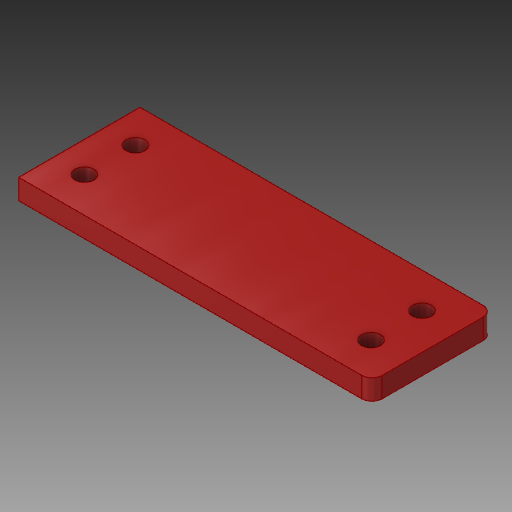
# Autodesk Inventor part: Gantry Chain Support
Saved by Autodesk Inventor 2019 (Build 230136000, 136)
## iProperties
Created: 2018-01-22
Part Number: Gantry Chain Support
Material: Steel
Document SubType Name: Modeling
Designer: torba
Density: 7.85 g/cm^3
Appearance: Red
Author: torba
Autodesk Inventor part; units mm, degrees
ref_plane "YZ Plane" through (0, 0, 0) normal (1, 0, 0) x (0, 1, 0)
ref_plane "XZ Plane" through (0, 0, 0) normal (0, 1, 0) x (-1, 0, 0)
ref_plane "XY Plane" through (0, 0, 0) normal (0, 0, 1) x (1, 0, 0)
sketch "Sketch1" plane through (0, 0, 0) normal (0, 1, 0) x (-1, 0, 0)
  circle A0 centre (-99.6006, 11.05) radius 3
  circle A1 centre (-9.6006, 11.05) radius 3
  circle A2 centre (-9.6006, 27.05) radius 3
  circle A3 centre (-99.6006, 27.05) radius 3
  arc A4 (-110.9506, 3.175) -> (-107.7756, 0) centre (-107.7756, 3.175) ccw
  line L0 (-107.7756, 0) -> (0, 0)
  line L1 (0, 38.1) -> (0, 0)
  line L2 (-107.7756, 38.1) -> (0, 38.1)
  arc A5 (-107.7756, 38.1) -> (-110.9506, 34.925) centre (-107.7756, 34.925) ccw
  line L3 (-110.9506, 3.175) -> (-110.9506, 34.925)
  point P0 (-62.2062, 0)
  dimension "d0" = 6
  dimension "d1" = 3.175
  dimension "d2" = 110.9506
  dimension "d3" = 38.1
  dimension "d4" = 0
  dimension "d5" = 38.1
  dimension "d6" = 9.6006
  dimension "d7" = 11.05
  dimension "d8" = 9.6006
  dimension "d9" = 27.05
  dimension "d10" = 62.2062
  dimension "d11" = 38.1
  dimension "d12" = 99.6006
  dimension "d13" = 11.05
  dimension "d14" = 99.6006
  dimension "d15" = 27.05
  constraints: 8 end point, 6 centre point, 4 equal radius, 4 point on circle, 4 tangent, 2 parallel, 1 horizontal, 1 vertical
  measures "d0" diameter of A2
  measures "d1" radius of A5
  measures "d2" distance between parallel lines of L1 L3
  measures "d3" distance between parallel lines of L2 L0
  measures "d4" distance from line of point (0, 0) L1
  measures "d5" distance from line of point (0, 0) L2
  measures "d6" distance from line of A2.centre L1
  measures "d7" distance from line of A2.centre L2
  measures "d8" distance from line of A1.centre L1
  measures "d9" distance from line of A1.centre L2
  measures "d10" distance from line of point (-62.206, 0) L1
  measures "d11" distance from line of point (-62.206, 0) L2
  measures "d12" distance from line of A3.centre L1
  measures "d13" distance from line of A3.centre L2
  measures "d14" distance from line of A0.centre L1
  measures "d15" distance from line of A0.centre L2
extrude "Extrusion1" add sketch "Sketch1" along normal blind 6.35
body "Solid1"
